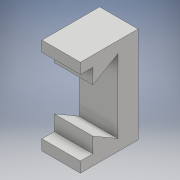
# Autodesk Inventor part: tester
Saved by Autodesk Inventor 2018 (Build 220112000, 112)
## iProperties
Created: 2018-09-13
Part Number: tester
Material: Generic
Document SubType Name: Modeling
Designer: David
Density: 1 g/cm^3
Appearance: Default
Author: David
Autodesk Inventor part; units mm, degrees
ref_plane "YZ Plane" through (0, 0, 0) normal (1, 0, 0) x (0, 1, 0)
ref_plane "XZ Plane" through (0, 0, 0) normal (0, 1, 0) x (-1, 0, 0)
ref_plane "XY Plane" through (0, 0, 0) normal (0, 0, 1) x (1, 0, 0)
sketch "Sketch1" plane through (0, 0, 0) normal (1, 0, 0) x (0, 1, 0)
  line L0 (-7.5, -12.5) -> (7.5, -12.5)
  line L1 (7.5, -12.5) -> (7.5, 12.5)
  line L2 (7.5, 12.5) -> (-7.5, 12.5)
  line L3 (-7.5, 12.5) -> (-7.5, -12.5)
  line L4 (-7.5, -12.5) -> (7.5, 12.5) construction
  line L5 (7.5, -12.5) -> (-7.5, 12.5) construction
  point P0 (0, 0)
  dimension "d0" = 25
  dimension "d1" = 15
  constraints: 12 end point, 2 midpoint, 2 parallel, 1 horizontal, 1 perpendicular
  measures "d0" distance of L0.end L1.end
  measures "d1" distance of L1.end L2.end
extrude "Extrusion1" add sketch "Sketch1" along normal blind 10
sketch "Sketch2" plane through (10, 0, 0) normal (1, 0, 0) x (0, 0, -1)
  line L0 (9.5, -4.5) -> (5.3472, -4.5) projected
  line L1 (9.5, -7.5) -> (9.5, -4.5) projected
  line L2 (9.5, -7.5) -> (22, -7.5) projected
  line L3 (22, 12.5) -> (22, -7.5) projected
  line L4 (-35, 12.5) -> (22, 12.5) projected
  line L5 (-35, 12.5) -> (-35, 59.5) projected
  line L6 (-45, 59.5) -> (-35, 59.5) projected
  line L7 (-45, 59.5) -> (-45, -7.5) projected
  line L8 (-45, -7.5) -> (-9.5, -7.5) projected
  line L9 (-9.5, -4.5) -> (-9.5, -7.5) projected
  line L10 (-5.3472, -4.5) -> (-9.5, -4.5) projected
  line L11 (-9.1, 2) -> (-5.3472, -4.5) projected
  line L12 (9.1, 2) -> (-9.1, 2) projected
  line L13 (5.3472, -4.5) -> (9.1, 2) projected
  line L14 (-9.5, -7.5) -> (9.5, -7.5)
  line L15 (-9.75, -7.25) -> (-44.75, -7.25)
  line L16 (-44.75, -7.25) -> (-44.75, 59.25)
  line L17 (-44.75, 59.25) -> (-35.25, 59.25)
  line L18 (-35.25, 59.25) -> (-35.25, 12.25)
  line L19 (-35.25, 12.25) -> (21.75, 12.25)
  line L20 (21.75, 12.25) -> (21.75, -7.25)
  line L21 (21.75, -7.25) -> (9.75, -7.25)
  line L22 (9.75, -7.25) -> (9.75, -4.25)
  line L23 (9.75, -4.25) -> (5.7802, -4.25)
  line L24 (5.7802, -4.25) -> (9.533, 2.25)
  line L25 (9.533, 2.25) -> (-9.533, 2.25)
  line L26 (-9.533, 2.25) -> (-5.7802, -4.25)
  line L27 (-5.7802, -4.25) -> (-9.75, -4.25)
  line L28 (-9.75, -4.25) -> (-9.75, -7.25)
  line L29 (-9.75, -7.25) -> (-9.75, -7.5)
  line L30 (-12.5, -7.5) -> (12.5, -7.5) projected
  line L31 (9.75, -7.25) -> (9.75, -7.5)
  line L32 (-12.5, -7.5) -> (12.5, -7.5) projected
  point P0 (0, 0)
  dimension "d4" = 0.25
  constraints: 34 end point, 3 perpendicular, 2 point on line, 13 other
  measures "d4" distance between parallel lines of L9 L28
extrude "Extrusion2" cut sketch "Sketch2" against normal blind 10 contours L1 L14 L9 L10 L11 L12 L13 L0 | L0 L13 L12 L11 L10 L9 L8 L29 L28 L27 L26 L25 L24 L23 L22 L31 L2 L1
body "Solid1"
